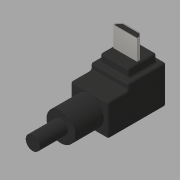
# Autodesk Inventor part: USB Micro Right Angle Plug
Saved by Autodesk Inventor 2019 (Build 230136000, 136)
## iProperties
Created: 2019-02-12
Part Number: USB Micro Right Angle Plug
Material: Generic
Document SubType Name: Modeling
Designer: Ben
Density: 1 g/cm^3
Appearance: Elec Black Plastic
Author: Ben
Autodesk Inventor part; units mm, degrees
ref_plane "YZ Plane" through (0, 0, 0) normal (1, 0, 0) x (0, 1, 0)
ref_plane "XZ Plane" through (0, 0, 0) normal (0, 1, 0) x (-1, 0, 0)
ref_plane "XY Plane" through (0, 0, 0) normal (0, 0, 1) x (1, 0, 0)
sketch "Sketch1" plane through (0, 0, 0) normal (0, 1, 0) x (-1, 0, 0)
  line L0 (-5.375, -8.25) -> (5.375, -8.25)
  line L1 (5.375, -8.25) -> (5.375, 8.25)
  line L2 (5.375, 8.25) -> (-5.375, 8.25)
  line L3 (-5.375, 8.25) -> (-5.375, -8.25)
  line L4 (-5.375, -8.25) -> (5.375, 8.25) construction
  line L5 (5.375, -8.25) -> (-5.375, 8.25) construction
  point P0 (0, 0)
  dimension "d0" = 10.75
  dimension "d1" = 16.5
  constraints: 12 end point, 2 midpoint, 2 parallel, 1 horizontal, 1 perpendicular
  measures "d0" distance of L2.end L1.end
  measures "d1" distance of L1.end L0.end
extrude "Extrusion1" add sketch "Sketch1" along normal blind 9
sketch "Sketch2" plane through (0, 9, 0) normal (0, 1, 0) x (1, 0, 0)
  line L0 (-5.375, 8.25) -> (-5.375, -8.25) projected
  line L1 (5.375, -8.25) -> (5.375, 8.25) projected
  line L2 (-5.375, 8.25) -> (5.375, 8.25)
  line L3 (5.375, 8.25) -> (5.375, -2.5)
  line L4 (5.375, -2.5) -> (-5.375, -2.5)
  line L5 (-5.375, -2.5) -> (-5.375, 8.25)
  point P0 (0, 0)
  dimension "d4" = 10.75
  constraints: 8 end point, 2 parallel, 1 horizontal, 1 perpendicular, 1 point on line
  measures "d4" distance of L2.end L3.end
extrude "Extrusion2" add sketch "Sketch2" along normal blind 1.75
sketch "Sketch3" plane through (0, 10.75, 0) normal (0, 1, 0) x (1, 0, 0)
  line L0 (5.375, 8.25) -> (-5.375, 8.25) construction
  line L1 (-5.375, 8.25) -> (-5.375, -2.5) construction
  line L2 (-5.375, -2.5) -> (5.375, -2.5) construction
  line L3 (5.375, -2.5) -> (5.375, 8.25) construction
  line L4 (5.375, 2.875) -> (-5.375, 2.875) construction
  line L5 (4, -1.125) -> (-4, -1.125)
  line L6 (-4, -1.125) -> (-4, 6.875)
  line L7 (-4, 6.875) -> (4, 6.875)
  line L8 (4, 6.875) -> (4, -1.125)
  line L9 (4, -1.125) -> (-4, 6.875) construction
  line L10 (-4, -1.125) -> (4, 6.875) construction
  point P0 (0, 0)
  point P1 (0, 2.875)
  dimension "d7" = 8
  dimension "d8" = 8
  constraints: 14 end point, 5 midpoint, 2 parallel, 1 horizontal, 1 perpendicular
  measures "d7" distance of L6.end L7.end
  measures "d8" distance of L5.end L6.end
extrude "Extrusion3" add sketch "Sketch3" along normal blind 2.33
fillet "Fillet1" radius 0.5 30 edges at (0, 13.08, 1.125) (-4, 13.08, -2.875) (0, 13.08, -6.875) (4, 13.08, -2.875) (4, 11.915, 1.125) (-4, 11.915, 1.125) (-4, 11.915, -6.875) (4, 11.915, -6.875) (0, 10.75, -6.875) (4, 10.75, -2.875) (0, 10.75, 1.125) (-4, 10.75, -2.875) (-5.375, 10.75, -2.875) (-5.375, 9.875, 2.5) (0, 10.75, 2.5) (5.375, 10.75, -2.875) (5.375, 9.875, 2.5) (5.375, 5.375, -8.25) (0, 10.75, -8.25) (-5.375, 5.375, -8.25) (-5.375, 9, 5.375) (5.375, 9, 5.375) (0, 9, 8.25) (5.375, 4.5, 8.25) (-5.375, 4.5, 8.25) (0, 0, 8.25) (5.375, 0, 0) (-5.375, 0, 0) (0, 0, -8.25) (0, 9, 2.5)
sketch "Sketch4" plane through (-4.875, 0.5, 8.25) normal (0, 0, 1) x (1, 0, 0)
  line L0 (9.75, 0) -> (0, 0) construction
  line L1 (9.75, 8) -> (9.75, 0) construction
  line L2 (0, 8) -> (9.75, 8) construction
  line L3 (0, 0) -> (0, 8) construction
  line L4 (0, 4) -> (9.75, 4) construction
  circle A0 centre (4.875, 4) radius 4.075
  point P0 (4.875, -0.5)
  dimension "d12" = 8.15
  constraints: 3 midpoint, 2 end point, 1 centre point
  measures "d12" diameter of A0
extrude "Extrusion4" add sketch "Sketch4" along normal blind 8.15
sketch "Sketch5" plane through (0, 13.08, 0) normal (0, 1, 0) x (1, 0, 0)
  line L0 (3.5, 6.375) -> (3.5, -0.625) construction
  line L1 (-3.5, 6.375) -> (3.5, 6.375) construction
  line L2 (-3.5, -0.625) -> (-3.5, 6.375) construction
  line L3 (3.5, -0.625) -> (-3.5, -0.625) construction
  line L4 (3.5, 2.875) -> (-3.5, 2.875) construction
  line L5 (3.4, 1.95) -> (-3.4, 1.95)
  line L6 (-3.4, 1.95) -> (-3.4, 3.8)
  line L7 (-3.4, 3.8) -> (3.4, 3.8)
  line L8 (3.4, 3.8) -> (3.4, 1.95)
  line L9 (3.4, 1.95) -> (-3.4, 3.8) construction
  line L10 (-3.4, 1.95) -> (3.4, 3.8) construction
  line L11 (2.4, 3.8) -> (3.4, 2.8)
  line L12 (-2.4, 3.8) -> (-3.4, 2.8)
  point P0 (0, 0)
  point P1 (0, 2.875)
  dimension "d15" = 6.8
  dimension "d16" = 1.85
  dimension "d17" = 0.85
  dimension "d18" = 1
  dimension "d19" = 1
  dimension "d20" = 0.85
  constraints: 18 end point, 5 midpoint, 4 point on line, 2 parallel, 1 horizontal, 1 perpendicular
  measures "d15" distance of L6.end L7.end
  measures "d16" distance of L5.end L6.end
  measures "d17" distance of L5.start L11.end
  measures "d18" distance of L7.end L11.start
  measures "d19" distance of L6.end L12.start
  measures "d20" distance of L5.end L12.end
extrude "Extrusion5" add sketch "Sketch5" along normal blind 5.75 separate body contours L5 L6 L12 L7 L11 L8
sketch "Sketch6" plane through (0, 18.83, 0) normal (0, 1, 0) x (1, 0, 0)
  line L0 (3.4, 1.95) -> (3.4, 2.8) construction
  line L1 (3.4, 2.8) -> (2.4, 3.8) construction
  line L2 (2.4, 3.8) -> (-2.4, 3.8) construction
  line L3 (-2.4, 3.8) -> (-3.4, 2.8) construction
  line L4 (-3.4, 2.8) -> (-3.4, 1.95) construction
  line L5 (-3.4, 1.95) -> (3.4, 1.95) construction
  line L6 (-2.3379, 3.65) -> (2.3379, 3.65)
  line L7 (2.3379, 3.65) -> (3.25, 2.7379)
  line L8 (3.25, 2.7379) -> (3.25, 2.1)
  line L9 (3.25, 2.1) -> (-3.25, 2.1)
  line L10 (-3.25, 2.1) -> (-3.25, 2.7379)
  line L11 (-3.25, 2.7379) -> (-2.3379, 3.65)
  point P0 (0, 0)
  dimension "d23" = 0.15
  constraints: 12 end point, 5 other
  measures "d23" distance between parallel lines of L2 L6
extrude "Extrusion6" cut sketch "Sketch6" against normal blind 0.15 bodies 2
sketch "Sketch7" plane through (0, 4.5, 16.4) normal (0, 0, 1) x (1, 0, 0)
  arc A0 (-0.7782, 4) -> (-0.7782, -4) centre (0, 0) ccw projected
  circle A1 centre (0, 0) radius 2
  point P0 (0, -4.5)
  dimension "d26" = 4
  constraints: 1 centre point, 1 coincident
  measures "d26" diameter of A1
extrude "Extrusion7" add sketch "Sketch7" along normal blind 8 bodies 1
equation "\"d4\" = d0"
body "Solid1"
body "Solid2"
